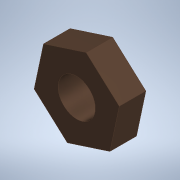
# Autodesk Inventor part: gaica
Saved by Autodesk Inventor 2021.2 (Build 252289000, 289)
## iProperties
Created: 2024-04-19
Part Number: gaica
Material: Bronze, Soft Tin
Document SubType Name: Modeling
Designer: cioba
Density: 8.874 g/cm^3
Appearance: Bronze - Satin
Author: cioba
Autodesk Inventor part; units mm, degrees
ref_plane "YZ Plane" through (0, 0, 0) normal (1, 0, 0) x (0, 1, 0)
ref_plane "XZ Plane" through (0, 0, 0) normal (0, 1, 0) x (-1, 0, 0)
ref_plane "XY Plane" through (0, 0, 0) normal (0, 0, 1) x (1, 0, 0)
sketch "Sketch1" plane through (0, 0, 0) normal (0, 0, 1) x (1, 0, 0)
  line L0 (4.0654, 27.1063) -> (2.3055, 18.8848)
  line L1 (2.3055, 18.8848) -> (-5.6945, 16.2981)
  line L2 (-5.6945, 16.2981) -> (-11.9346, 21.933)
  line L3 (-11.9346, 21.933) -> (-10.1748, 30.1545)
  line L4 (-10.1748, 30.1545) -> (-2.1748, 32.7412)
  line L5 (-2.1748, 32.7412) -> (4.0654, 27.1063)
  circle A0 centre (-3.9346, 24.5196) radius 3.5
  constraints: 12 end point, 1 centre point, 1 coincident, 13 other
extrude "Extrusion4" add sketch "Sketch1" against normal blind 5
body "Solid2"
